Autodesk Inventor part; units mm, degrees
(part 2 of 3)
  line L944 (16.9524, -6.6944) -> (16.9314, -6.7061)
  line L945 (16.9314, -6.7061) -> (16.9218, -6.7147)
  line L946 (16.9218, -6.7147) -> (16.9143, -6.7266)
  line L947 (16.9143, -6.7266) -> (16.909, -6.7418)
  line L948 (16.909, -6.7418) -> (16.906, -6.76)
  line L949 (16.906, -6.76) -> (16.9054, -6.7813)
  line L950 (16.9054, -6.7813) -> (16.9073, -6.8056)
  line L951 (16.9073, -6.8056) -> (16.912, -6.8327)
  line L952 (16.912, -6.8327) -> (16.9194, -6.8625)
  line L953 (16.9194, -6.8625) -> (16.9472, -6.9448)
  line L954 (16.9472, -6.9448) -> (16.9649, -7.0024)
  line L955 (16.9649, -7.0024) -> (16.9847, -7.0784)
  line L956 (16.9847, -7.0784) -> (17.0036, -7.1659)
  line L957 (17.0036, -7.1659) -> (17.0214, -7.2683)
  line L958 (17.0214, -7.2683) -> (17.0364, -7.3838)
  line L959 (17.0364, -7.3838) -> (17.0479, -7.5139)
  line L960 (17.0479, -7.5139) -> (17.0545, -7.6588)
  line L961 (17.0545, -7.6588) -> (17.0557, -7.7357)
  line L962 (17.0557, -7.7357) -> (17.0536, -7.88)
  arc A25 (16.7145, -8.0349) -> (17.0536, -7.88) centre (13.25, 0) ccw
  line L963 (16.7145, -8.0349) -> (16.6041, -7.942)
  line L964 (16.6041, -7.942) -> (16.5467, -7.8907)
  line L965 (16.5467, -7.8907) -> (16.4415, -7.7908)
  line L966 (16.4415, -7.7908) -> (16.3508, -7.697)
  line L967 (16.3508, -7.697) -> (16.2733, -7.6099)
  line L968 (16.2733, -7.6099) -> (16.2075, -7.5295)
  line L969 (16.2075, -7.5295) -> (16.1538, -7.4579)
  line L970 (16.1538, -7.4579) -> (16.1094, -7.3931)
  line L971 (16.1094, -7.3931) -> (16.0773, -7.342)
  line L972 (16.0773, -7.342) -> (16.0334, -7.2672)
  line L973 (16.0334, -7.2672) -> (16.0157, -7.242)
  line L974 (16.0157, -7.242) -> (15.9983, -7.2207)
  line L975 (15.9983, -7.2207) -> (15.9812, -7.2034)
  line L976 (15.9812, -7.2034) -> (15.9647, -7.1899)
  line L977 (15.9647, -7.1899) -> (15.949, -7.1802)
  line L978 (15.949, -7.1802) -> (15.934, -7.1743)
  line L979 (15.934, -7.1743) -> (15.9201, -7.1722)
  line L980 (15.9201, -7.1722) -> (15.9073, -7.1738)
  line L981 (15.9073, -7.1738) -> (15.8847, -7.182)
  line L982 (15.8847, -7.182) -> (15.7521, -7.2293)
  line L983 (15.7521, -7.2293) -> (15.6186, -7.2741)
  line L984 (15.6186, -7.2741) -> (15.5957, -7.2816)
  line L985 (15.5957, -7.2816) -> (15.5847, -7.2883)
  line L986 (15.5847, -7.2883) -> (15.5751, -7.2986)
  line L987 (15.5751, -7.2986) -> (15.567, -7.3124)
  line L988 (15.567, -7.3124) -> (15.5605, -7.3298)
  line L989 (15.5605, -7.3298) -> (15.5559, -7.3506)
  line L990 (15.5559, -7.3506) -> (15.5533, -7.3747)
  line L991 (15.5533, -7.3747) -> (15.5527, -7.4022)
  line L992 (15.5527, -7.4022) -> (15.5544, -7.433)
  line L993 (15.5544, -7.433) -> (15.5661, -7.519)
  line L994 (15.5661, -7.519) -> (15.5725, -7.5789)
  line L995 (15.5725, -7.5789) -> (15.5776, -7.6573)
  line L996 (15.5776, -7.6573) -> (15.5796, -7.7468)
  line L997 (15.5796, -7.7468) -> (15.5777, -7.8506)
  line L998 (15.5777, -7.8506) -> (15.5706, -7.967)
  line L999 (15.5706, -7.967) -> (15.5572, -8.0968)
  line L1000 (15.5572, -8.0968) -> (15.5364, -8.2404)
  line L1001 (15.5364, -8.2404) -> (15.5229, -8.3162)
  line L1002 (15.5229, -8.3162) -> (15.4935, -8.4575)
  arc A26 (15.1313, -8.5454) -> (15.4935, -8.4575) centre (13.25, 0) ccw
  line L1003 (15.1313, -8.5454) -> (15.0404, -8.4332)
  line L1004 (15.0404, -8.4332) -> (14.9938, -8.372)
  line L1005 (14.9938, -8.372) -> (14.9094, -8.254)
  line L1006 (14.9094, -8.254) -> (14.8381, -8.1447)
  line L1007 (14.8381, -8.1447) -> (14.7785, -8.0445)
  line L1008 (14.7785, -8.0445) -> (14.7291, -7.9531)
  line L1009 (14.7291, -7.9531) -> (14.6899, -7.8727)
  line L1010 (14.6899, -7.8727) -> (14.6585, -7.8006)
  line L1011 (14.6585, -7.8006) -> (14.6368, -7.7444)
  line L1012 (14.6368, -7.7444) -> (14.6078, -7.6626)
  line L1013 (14.6078, -7.6626) -> (14.5952, -7.6345)
  line L1014 (14.5952, -7.6345) -> (14.5821, -7.6104)
  line L1015 (14.5821, -7.6104) -> (14.5686, -7.5901)
  line L1016 (14.5686, -7.5901) -> (14.555, -7.5737)
  line L1017 (14.555, -7.5737) -> (14.5413, -7.5612)
  line L1018 (14.5413, -7.5612) -> (14.5278, -7.5526)
  line L1019 (14.5278, -7.5526) -> (14.5145, -7.5479)
  line L1020 (14.5145, -7.5479) -> (14.5017, -7.547)
  line L1021 (14.5017, -7.547) -> (14.4779, -7.5508)
  line L1022 (14.4779, -7.5508) -> (14.3387, -7.5721)
  line L1023 (14.3387, -7.5721) -> (14.1992, -7.5909)
  line L1024 (14.1992, -7.5909) -> (14.1753, -7.594)
  line L1025 (14.1753, -7.594) -> (14.1632, -7.5984)
  line L1026 (14.1632, -7.5984) -> (14.1518, -7.6067)
  line L1027 (14.1518, -7.6067) -> (14.1412, -7.6187)
  line L1028 (14.1412, -7.6187) -> (14.1316, -7.6346)
  line L1029 (14.1316, -7.6346) -> (14.1232, -7.6541)
  line L1030 (14.1232, -7.6541) -> (14.116, -7.6774)
  line L1031 (14.116, -7.6774) -> (14.1102, -7.7043)
  line L1032 (14.1102, -7.7043) -> (14.106, -7.7347)
  line L1033 (14.106, -7.7347) -> (14.1013, -7.8214)
  line L1034 (14.1013, -7.8214) -> (14.0962, -7.8815)
  line L1035 (14.0962, -7.8815) -> (14.0864, -7.9594)
  line L1036 (14.0864, -7.9594) -> (14.0714, -8.0477)
  line L1037 (14.0714, -8.0477) -> (14.0499, -8.1493)
  line L1038 (14.0499, -8.1493) -> (14.0209, -8.2622)
  line L1039 (14.0209, -8.2622) -> (13.9832, -8.3872)
  line L1040 (13.9832, -8.3872) -> (13.9355, -8.5242)
  line L1041 (13.9355, -8.5242) -> (13.908, -8.5961)
  line L1042 (13.908, -8.5961) -> (13.8524, -8.7292)
  arc A27 (13.4801, -8.747) -> (13.8524, -8.7292) centre (13.25, 0) ccw
  line L1043 (13.4801, -8.747) -> (13.4121, -8.6197)
  line L1044 (13.4121, -8.6197) -> (13.3778, -8.5507)
  line L1045 (13.3778, -8.5507) -> (13.3174, -8.4189)
  line L1046 (13.3174, -8.4189) -> (13.268, -8.2981)
  line L1047 (13.268, -8.2981) -> (13.2284, -8.1884)
  line L1048 (13.2284, -8.1884) -> (13.1973, -8.0893)
  line L1049 (13.1973, -8.0893) -> (13.174, -8.0029)
  line L1050 (13.174, -8.0029) -> (13.1568, -7.9262)
  line L1051 (13.1568, -7.9262) -> (13.1461, -7.8669)
  line L1052 (13.1461, -7.8669) -> (13.1331, -7.7811)
  line L1053 (13.1331, -7.7811) -> (13.126, -7.7511)
  line L1054 (13.126, -7.7511) -> (13.1177, -7.7249)
  line L1055 (13.1177, -7.7249) -> (13.1084, -7.7025)
  line L1056 (13.1084, -7.7025) -> (13.0981, -7.6838)
  line L1057 (13.0981, -7.6838) -> (13.087, -7.669)
  line L1058 (13.087, -7.669) -> (13.0753, -7.658)
  line L1059 (13.0753, -7.658) -> (13.0632, -7.6508)
  line L1060 (13.0632, -7.6508) -> (13.0508, -7.6475)
  line L1061 (13.0508, -7.6475) -> (13.0267, -7.6468)
  line L1062 (13.0267, -7.6468) -> (12.886, -7.6413)
  line L1063 (12.886, -7.6413) -> (12.7454, -7.6334)
  line L1064 (12.7454, -7.6334) -> (12.7214, -7.6318)
  line L1065 (12.7214, -7.6318) -> (12.7087, -7.6339)
  line L1066 (12.7087, -7.6339) -> (12.6959, -7.6399)
  line L1067 (12.6959, -7.6399) -> (12.6833, -7.6497)
  line L1068 (12.6833, -7.6497) -> (12.6708, -7.6635)
  line L1069 (12.6708, -7.6635) -> (12.6588, -7.6811)
  line L1070 (12.6588, -7.6811) -> (12.6474, -7.7025)
  line L1071 (12.6474, -7.7025) -> (12.6366, -7.7278)
  line L1072 (12.6366, -7.7278) -> (12.6267, -7.757)
  line L1073 (12.6267, -7.757) -> (12.6057, -7.8412)
  line L1074 (12.6057, -7.8412) -> (12.5893, -7.8992)
  line L1075 (12.5893, -7.8992) -> (12.5649, -7.9739)
  line L1076 (12.5649, -7.9739) -> (12.5336, -8.0577)
  line L1077 (12.5336, -8.0577) -> (12.4931, -8.1534)
  line L1078 (12.4931, -8.1534) -> (12.4433, -8.2588)
  line L1079 (12.4433, -8.2588) -> (12.3827, -8.3744)
  line L1080 (12.3827, -8.3744) -> (12.3099, -8.4999)
  line L1081 (12.3099, -8.4999) -> (12.2693, -8.5652)
  line L1082 (12.2693, -8.5652) -> (12.1895, -8.6855)
  arc A28 (11.8205, -8.6324) -> (12.1895, -8.6855) centre (13.25, 0) ccw
  line L1083 (11.8205, -8.6324) -> (11.7779, -8.4946)
  line L1084 (11.7779, -8.4946) -> (11.7573, -8.4204)
  line L1085 (11.7573, -8.4204) -> (11.7229, -8.2795)
  line L1086 (11.7229, -8.2795) -> (11.6972, -8.1515)
  line L1087 (11.6972, -8.1515) -> (11.6791, -8.0364)
  line L1088 (11.6791, -8.0364) -> (11.6673, -7.9332)
  line L1089 (11.6673, -7.9332) -> (11.6608, -7.8439)
  line L1090 (11.6608, -7.8439) -> (11.6584, -7.7654)
  line L1091 (11.6584, -7.7654) -> (11.6591, -7.7051)
  line L1092 (11.6591, -7.7051) -> (11.6626, -7.6183)
  line L1093 (11.6626, -7.6183) -> (11.6614, -7.5876)
  line L1094 (11.6614, -7.5876) -> (11.6582, -7.5603)
  line L1095 (11.6582, -7.5603) -> (11.6532, -7.5365)
  line L1096 (11.6532, -7.5365) -> (11.6467, -7.5162)
  line L1097 (11.6467, -7.5162) -> (11.6386, -7.4995)
  line L1098 (11.6386, -7.4995) -> (11.6292, -7.4865)
  line L1099 (11.6292, -7.4865) -> (11.6187, -7.4772)
  line L1100 (11.6187, -7.4772) -> (11.6071, -7.4716)
  line L1101 (11.6071, -7.4716) -> (11.5836, -7.4663)
  line L1102 (11.5836, -7.4663) -> (11.4464, -7.4344)
  line L1103 (11.4464, -7.4344) -> (11.3099, -7.3999)
  line L1104 (11.3099, -7.3999) -> (11.2866, -7.3939)
  line L1105 (11.2866, -7.3939) -> (11.2737, -7.3935)
  line L1106 (11.2737, -7.3935) -> (11.2601, -7.397)
  line L1107 (11.2601, -7.397) -> (11.2458, -7.4042)
  line L1108 (11.2458, -7.4042) -> (11.231, -7.4154)
  line L1109 (11.231, -7.4154) -> (11.2159, -7.4304)
  line L1110 (11.2159, -7.4304) -> (11.2005, -7.4493)
  line L1111 (11.2005, -7.4493) -> (11.1852, -7.4721)
  line L1112 (11.1852, -7.4721) -> (11.17, -7.4988)
  line L1113 (11.17, -7.4988) -> (11.1334, -7.5775)
  line L1114 (11.1334, -7.5775) -> (11.1063, -7.6314)
  line L1115 (11.1063, -7.6314) -> (11.0683, -7.7001)
  line L1116 (11.0683, -7.7001) -> (11.0216, -7.7765)
  line L1117 (11.0216, -7.7765) -> (10.9638, -7.8628)
  line L1118 (10.9638, -7.8628) -> (10.8949, -7.9569)
  line L1119 (10.8949, -7.9569) -> (10.8135, -8.0589)
  line L1120 (10.8135, -8.0589) -> (10.7183, -8.1683)
  line L1121 (10.7183, -8.1683) -> (10.666, -8.2249)
  line L1122 (10.666, -8.2249) -> (10.5649, -8.3278)
  arc A29 (10.2127, -8.2059) -> (10.5649, -8.3278) centre (13.25, 0) ccw
  line L1123 (10.2127, -8.2059) -> (10.1969, -8.0625)
  line L1124 (10.1969, -8.0625) -> (10.1907, -7.9857)
  line L1125 (10.1907, -7.9857) -> (10.1836, -7.8409)
  line L1126 (10.1836, -7.8409) -> (10.1826, -7.7103)
  line L1127 (10.1826, -7.7103) -> (10.1866, -7.5938)
  line L1128 (10.1866, -7.5938) -> (10.1945, -7.4903)
  line L1129 (10.1945, -7.4903) -> (10.2051, -7.4014)
  line L1130 (10.2051, -7.4014) -> (10.2176, -7.3238)
  line L1131 (10.2176, -7.3238) -> (10.2297, -7.2647)
  line L1132 (10.2297, -7.2647) -> (10.2495, -7.1803)
  line L1133 (10.2495, -7.1803) -> (10.2541, -7.1498)
  line L1134 (10.2541, -7.1498) -> (10.2561, -7.1224)
  line L1135 (10.2561, -7.1224) -> (10.2558, -7.0981)
  line L1136 (10.2558, -7.0981) -> (10.2532, -7.0769)
  line L1137 (10.2532, -7.0769) -> (10.2484, -7.059)
  line L1138 (10.2484, -7.059) -> (10.2417, -7.0445)
  line L1139 (10.2417, -7.0445) -> (10.2331, -7.0333)
  line L1140 (10.2331, -7.0333) -> (10.2227, -7.0257)
  line L1141 (10.2227, -7.0257) -> (10.2007, -7.016)
  line L1142 (10.2007, -7.016) -> (10.0721, -6.9587)
  line L1143 (10.0721, -6.9587) -> (9.9445, -6.899)
  line L1144 (9.9445, -6.899) -> (9.9228, -6.8887)
  line L1145 (9.9228, -6.8887) -> (9.9102, -6.8859)
  line L1146 (9.9102, -6.8859) -> (9.8962, -6.8867)
  line L1147 (9.8962, -6.8867) -> (9.8807, -6.8911)
  line L1148 (9.8807, -6.8911) -> (9.8641, -6.8993)
  line L1149 (9.8641, -6.8993) -> (9.8464, -6.9111)
  line L1150 (9.8464, -6.9111) -> (9.8278, -6.9268)
  line L1151 (9.8278, -6.9268) -> (9.8084, -6.9463)
  line L1152 (9.8084, -6.9463) -> (9.7884, -6.9697)
  line L1153 (9.7884, -6.9697) -> (9.7376, -7.04)
  line L1154 (9.7376, -7.04) -> (9.7008, -7.0878)
  line L1155 (9.7008, -7.0878) -> (9.6504, -7.1481)
  line L1156 (9.6504, -7.1481) -> (9.5901, -7.2143)
  line L1157 (9.5901, -7.2143) -> (9.5171, -7.2881)
  line L1158 (9.5171, -7.2881) -> (9.4316, -7.3674)
  line L1159 (9.4316, -7.3674) -> (9.3324, -7.4521)
  line L1160 (9.3324, -7.4521) -> (9.2182, -7.5416)
  line L1161 (9.2182, -7.5416) -> (9.1562, -7.5872)
  line L1162 (9.1562, -7.5872) -> (9.0374, -7.6692)
  arc A30 (8.7146, -7.4828) -> (9.0374, -7.6692) centre (13.25, 0) ccw
  line L1163 (8.7146, -7.4828) -> (8.7262, -7.339)
  line L1164 (8.7262, -7.339) -> (8.7347, -7.2624)
  line L1165 (8.7347, -7.2624) -> (8.7551, -7.1188)
  line L1166 (8.7551, -7.1188) -> (8.7788, -6.9905)
  line L1167 (8.7788, -6.9905) -> (8.8048, -6.8769)
  line L1168 (8.8048, -6.8769) -> (8.8322, -6.7767)
  line L1169 (8.8322, -6.7767) -> (8.8594, -6.6914)
  line L1170 (8.8594, -6.6914) -> (8.8863, -6.6176)
  line L1171 (8.8863, -6.6176) -> (8.9094, -6.5619)
  line L1172 (8.9094, -6.5619) -> (8.9449, -6.4827)
  line L1173 (8.9449, -6.4827) -> (8.9551, -6.4536)
  line L1174 (8.9551, -6.4536) -> (8.9623, -6.4271)
  line L1175 (8.9623, -6.4271) -> (8.9666, -6.4032)
  line L1176 (8.9666, -6.4032) -> (8.968, -6.3819)
  line L1177 (8.968, -6.3819) -> (8.9667, -6.3634)
  line L1178 (8.9667, -6.3634) -> (8.9629, -6.3479)
  line L1179 (8.9629, -6.3479) -> (8.9565, -6.3353)
  line L1180 (8.9565, -6.3353) -> (8.9478, -6.3258)
  line L1181 (8.9478, -6.3258) -> (8.928, -6.3121)
  line L1182 (8.928, -6.3121) -> (8.8126, -6.2315)
  line L1183 (8.8126, -6.2315) -> (8.6986, -6.1488)
  line L1184 (8.6986, -6.1488) -> (8.6792, -6.1345)
  line L1185 (8.6792, -6.1345) -> (8.6674, -6.1294)
  line L1186 (8.6674, -6.1294) -> (8.6535, -6.1275)
  line L1187 (8.6535, -6.1275) -> (8.6375, -6.129)
  line L1188 (8.6375, -6.129) -> (8.6196, -6.1338)
  line L1189 (8.6196, -6.1338) -> (8.6, -6.1421)
  line L1190 (8.6, -6.1421) -> (8.5787, -6.154)
  line L1191 (8.5787, -6.154) -> (8.556, -6.1694)
  line L1192 (8.556, -6.1694) -> (8.532, -6.1886)
  line L1193 (8.532, -6.1886) -> (8.4687, -6.248)
  line L1194 (8.4687, -6.248) -> (8.4236, -6.2881)
  line L1195 (8.4236, -6.2881) -> (8.3627, -6.3377)
  line L1196 (8.3627, -6.3377) -> (8.291, -6.3913)
  line L1197 (8.291, -6.3913) -> (8.2052, -6.4499)
  line L1198 (8.2052, -6.4499) -> (8.1063, -6.5116)
  line L1199 (8.1063, -6.5116) -> (7.9928, -6.576)
  line L1200 (7.9928, -6.576) -> (7.8638, -6.6423)
  line L1201 (7.8638, -6.6423) -> (7.7943, -6.6753)
  line L1202 (7.7943, -6.6753) -> (7.6621, -6.7334)
  arc A31 (7.3804, -6.4893) -> (7.6621, -6.7334) centre (13.25, 0) ccw
  line L1203 (7.3804, -6.4893) -> (7.4191, -6.3502)
  line L1204 (7.4191, -6.3502) -> (7.4418, -6.2767)
  line L1205 (7.4418, -6.2767) -> (7.4891, -6.1395)
  line L1206 (7.4891, -6.1395) -> (7.5367, -6.018)
  line L1207 (7.5367, -6.018) -> (7.5837, -5.9113)
  line L1208 (7.5837, -5.9113) -> (7.6295, -5.8181)
  line L1209 (7.6295, -5.8181) -> (7.6724, -5.7395)
  line L1210 (7.6724, -5.7395) -> (7.7128, -5.6722)
  line L1211 (7.7128, -5.6722) -> (7.746, -5.6218)
  line L1212 (7.746, -5.6218) -> (7.7958, -5.5508)
  line L1213 (7.7958, -5.5508) -> (7.8114, -5.5242)
  line L1214 (7.8114, -5.5242) -> (7.8235, -5.4995)
  line L1215 (7.8235, -5.4995) -> (7.8322, -5.4768)
  line L1216 (7.8322, -5.4768) -> (7.8376, -5.4562)
  line L1217 (7.8376, -5.4562) -> (7.8399, -5.4378)
  line L1218 (7.8399, -5.4378) -> (7.839, -5.4218)
  line L1219 (7.839, -5.4218) -> (7.8352, -5.4082)
  line L1220 (7.8352, -5.4082) -> (7.8284, -5.3973)
  line L1221 (7.8284, -5.3973) -> (7.8115, -5.3801)
  line L1222 (7.8115, -5.3801) -> (7.7134, -5.2791)
  line L1223 (7.7134, -5.2791) -> (7.6172, -5.1763)
  line L1224 (7.6172, -5.1763) -> (7.6008, -5.1586)
  line L1225 (7.6008, -5.1586) -> (7.5902, -5.1514)
  line L1226 (7.5902, -5.1514) -> (7.5769, -5.1469)
  line L1227 (7.5769, -5.1469) -> (7.5609, -5.1453)
  line L1228 (7.5609, -5.1453) -> (7.5424, -5.1466)
  line L1229 (7.5424, -5.1466) -> (7.5216, -5.1511)
  line L1230 (7.5216, -5.1511) -> (7.4985, -5.1587)
  line L1231 (7.4985, -5.1587) -> (7.4733, -5.1696)
  line L1232 (7.4733, -5.1696) -> (7.446, -5.1839)
  line L1233 (7.446, -5.1839) -> (7.3727, -5.2303)
  line L1234 (7.3727, -5.2303) -> (7.3208, -5.261)
  line L1235 (7.3208, -5.261) -> (7.2516, -5.2982)
  line L1236 (7.2516, -5.2982) -> (7.171, -5.3373)
  line L1237 (7.171, -5.3373) -> (7.0758, -5.3786)
  line L1238 (7.0758, -5.3786) -> (6.967, -5.4205)
  line L1239 (6.967, -5.4205) -> (6.8433, -5.4623)
  line L1240 (6.8433, -5.4623) -> (6.7041, -5.5029)
  line L1241 (6.7041, -5.5029) -> (6.6295, -5.5222)
  line L1242 (6.6295, -5.5222) -> (6.4888, -5.5542)
  arc A32 (6.2584, -5.2612) -> (6.4888, -5.5542) centre (13.25, 0) ccw
  line L1243 (6.2584, -5.2612) -> (6.3226, -5.1319)
  line L1244 (6.3226, -5.1319) -> (6.3589, -5.064)
  line L1245 (6.3589, -5.064) -> (6.4313, -4.9383)
  line L1246 (6.4313, -4.9383) -> (6.501, -4.828)
  line L1247 (6.501, -4.828) -> (6.5674, -4.7321)
  line L1248 (6.5674, -4.7321) -> (6.63, -4.6493)
  line L1249 (6.63, -4.6493) -> (6.6869, -4.5802)
  line L1250 (6.6869, -4.5802) -> (6.7394, -4.5218)
  line L1251 (6.7394, -4.5218) -> (6.7815, -4.4786)
  line L1252 (6.7815, -4.4786) -> (6.8439, -4.4182)
  line L1253 (6.8439, -4.4182) -> (6.8642, -4.3951)
  line L1254 (6.8642, -4.3951) -> (6.8807, -4.3732)
  line L1255 (6.8807, -4.3732) -> (6.8936, -4.3525)
  line L1256 (6.8936, -4.3525) -> (6.9028, -4.3333)
  line L1257 (6.9028, -4.3333) -> (6.9085, -4.3157)
  line L1258 (6.9085, -4.3157) -> (6.9107, -4.2998)
  line L1259 (6.9107, -4.2998) -> (6.9095, -4.2857)
  line L1260 (6.9095, -4.2857) -> (6.9049, -4.2737)
  line L1261 (6.9049, -4.2737) -> (6.8916, -4.2537)
  line L1262 (6.8916, -4.2537) -> (6.8144, -4.1359)
  line L1263 (6.8144, -4.1359) -> (6.7394, -4.0168)
  line L1264 (6.7394, -4.0168) -> (6.7267, -3.9963)
  line L1265 (6.7267, -3.9963) -> (6.7176, -3.9872)
  line L1266 (6.7176, -3.9872) -> (6.7053, -3.9802)
  line L1267 (6.7053, -3.9802) -> (6.69, -3.9756)
  line L1268 (6.69, -3.9756) -> (6.6716, -3.9735)
  line L1269 (6.6716, -3.9735) -> (6.6503, -3.9739)
  line L1270 (6.6503, -3.9739) -> (6.6262, -3.977)
  line L1271 (6.6262, -3.977) -> (6.5993, -3.9829)
  line L1272 (6.5993, -3.9829) -> (6.5698, -3.9918)
  line L1273 (6.5698, -3.9918) -> (6.489, -4.0235)
  line L1274 (6.489, -4.0235) -> (6.4323, -4.0438)
  line L1275 (6.4323, -4.0438) -> (6.3573, -4.0673)
  line L1276 (6.3573, -4.0673) -> (6.2708, -4.0904)
  line L1277 (6.2708, -4.0904) -> (6.1694, -4.1129)
  line L1278 (6.1694, -4.1129) -> (6.0547, -4.1335)
  line L1279 (6.0547, -4.1335) -> (5.9254, -4.1511)
  line L1280 (5.9254, -4.1511) -> (5.7809, -4.1647)
  line L1281 (5.7809, -4.1647) -> (5.7041, -4.1695)
  line L1282 (5.7041, -4.1695) -> (5.5599, -4.1742)
  arc A33 (5.3891, -3.8429) -> (5.5599, -4.1742) centre (13.25, 0) ccw
  line L1283 (5.3891, -3.8429) -> (5.4766, -3.7282)
  line L1284 (5.4766, -3.7282) -> (5.5251, -3.6684)
  line L1285 (5.5251, -3.6684) -> (5.6199, -3.5586)
  line L1286 (5.6199, -3.5586) -> (5.7093, -3.4635)
  line L1287 (5.7093, -3.4635) -> (5.7926, -3.3819)
  line L1288 (5.7926, -3.3819) -> (5.8698, -3.3125)
  line L1289 (5.8698, -3.3125) -> (5.9387, -3.2554)
  line L1290 (5.9387, -3.2554) -> (6.0013, -3.2079)
  line L1291 (6.0013, -3.2079) -> (6.0508, -3.1735)
  line L1292 (6.0508, -3.1735) -> (6.1235, -3.126)
  line L1293 (6.1235, -3.126) -> (6.1478, -3.1072)
  line L1294 (6.1478, -3.1072) -> (6.1682, -3.0887)
  line L1295 (6.1682, -3.0887) -> (6.1847, -3.0709)
  line L1296 (6.1847, -3.0709) -> (6.1974, -3.0538)
  line L1297 (6.1974, -3.0538) -> (6.2064, -3.0375)
  line L1298 (6.2064, -3.0375) -> (6.2115, -3.0223)
  line L1299 (6.2115, -3.0223) -> (6.213, -3.0083)
  line L1300 (6.213, -3.0083) -> (6.2108, -2.9957)
  line L1301 (6.2108, -2.9957) -> (6.2015, -2.9735)
  line L1302 (6.2015, -2.9735) -> (6.148, -2.8432)
  line L1303 (6.148, -2.8432) -> (6.0968, -2.712)
  line L1304 (6.0968, -2.712) -> (6.0882, -2.6895)
  line L1305 (6.0882, -2.6895) -> (6.0811, -2.6789)
  line L1306 (6.0811, -2.6789) -> (6.0703, -2.6697)
  line L1307 (6.0703, -2.6697) -> (6.0561, -2.6623)
  line L1308 (6.0561, -2.6623) -> (6.0385, -2.6567)
  line L1309 (6.0385, -2.6567) -> (6.0175, -2.6531)
  line L1310 (6.0175, -2.6531) -> (5.9932, -2.6516)
  line L1311 (5.9932, -2.6516) -> (5.9657, -2.6523)
  line L1312 (5.9657, -2.6523) -> (5.9351, -2.6554)
  line L1313 (5.9351, -2.6554) -> (5.8498, -2.6712)
  line L1314 (5.8498, -2.6712) -> (5.7902, -2.6805)
  line L1315 (5.7902, -2.6805) -> (5.7121, -2.6893)
  line L1316 (5.7121, -2.6893) -> (5.6228, -2.6956)
  line L1317 (5.6228, -2.6956) -> (5.519, -2.6986)
  line L1318 (5.519, -2.6986) -> (5.4024, -2.697)
  line L1319 (5.4024, -2.697) -> (5.2721, -2.6899)
  line L1320 (5.2721, -2.6899) -> (5.1277, -2.6759)
  line L1321 (5.1277, -2.6759) -> (5.0514, -2.666)
  line L1322 (5.0514, -2.666) -> (4.9089, -2.6434)
  arc A34 (4.8038, -2.2858) -> (4.9089, -2.6434) centre (13.25, 0) ccw
  line L1323 (4.8038, -2.2858) -> (4.9115, -2.1897)
  line L1324 (4.9115, -2.1897) -> (4.9704, -2.1401)
  line L1325 (4.9704, -2.1401) -> (5.0843, -2.0503)
  line L1326 (5.0843, -2.0503) -> (5.1901, -1.9738)
  line L1327 (5.1901, -1.9738) -> (5.2873, -1.9095)
  line L1328 (5.2873, -1.9095) -> (5.3762, -1.8559)
  line L1329 (5.3762, -1.8559) -> (5.4548, -1.8129)
  line L1330 (5.4548, -1.8129) -> (5.5252, -1.7781)
  line L1331 (5.5252, -1.7781) -> (5.5804, -1.7537)
  line L1332 (5.5804, -1.7537) -> (5.6607, -1.7208)
  line L1333 (5.6607, -1.7208) -> (5.6881, -1.7069)
  line L1334 (5.6881, -1.7069) -> (5.7116, -1.6927)
  line L1335 (5.7116, -1.6927) -> (5.7313, -1.6783)
  line L1336 (5.7313, -1.6783) -> (5.747, -1.6639)
  line L1337 (5.747, -1.6639) -> (5.7588, -1.6496)
  line L1338 (5.7588, -1.6496) -> (5.7667, -1.6357)
  line L1339 (5.7667, -1.6357) -> (5.7708, -1.6222)
  line L1340 (5.7708, -1.6222) -> (5.7711, -1.6094)
  line L1341 (5.7711, -1.6094) -> (5.7661, -1.5858)
  line L1342 (5.7661, -1.5858) -> (5.7382, -1.4478)
  line L1343 (5.7382, -1.4478) -> (5.7128, -1.3093)
  line L1344 (5.7128, -1.3093) -> (5.7087, -1.2856)
  line L1345 (5.7087, -1.2856) -> (5.7036, -1.2737)
  line L1346 (5.7036, -1.2737) -> (5.6948, -1.2627)
  line L1347 (5.6948, -1.2627) -> (5.6823, -1.2527)
  line L1348 (5.6823, -1.2527) -> (5.666, -1.2439)
  line L1349 (5.666, -1.2439) -> (5.6461, -1.2364)
  line L1350 (5.6461, -1.2364) -> (5.6225, -1.2303)
  line L1351 (5.6225, -1.2303) -> (5.5954, -1.2258)
  line L1352 (5.5954, -1.2258) -> (5.5648, -1.2231)
  line L1353 (5.5648, -1.2231) -> (5.478, -1.2224)
  line L1354 (5.478, -1.2224) -> (5.4177, -1.2203)
  line L1355 (5.4177, -1.2203) -> (5.3394, -1.2142)
  line L1356 (5.3394, -1.2142) -> (5.2505, -1.2034)
  line L1357 (5.2505, -1.2034) -> (5.148, -1.1867)
  line L1358 (5.148, -1.1867) -> (5.0338, -1.1631)
  line L1359 (5.0338, -1.1631) -> (4.9072, -1.1315)
  line L1360 (4.9072, -1.1315) -> (4.7681, -1.0904)
  line L1361 (4.7681, -1.0904) -> (4.695, -1.0663)
  line L1362 (4.695, -1.0663) -> (4.5593, -1.0171)
  arc A35 (4.5239, -0.646) -> (4.5593, -1.0171) centre (13.25, 0) ccw
  line L1363 (4.5239, -0.646) -> (4.6478, -0.572)
  line L1364 (4.6478, -0.572) -> (4.715, -0.5346)
  line L1365 (4.715, -0.5346) -> (4.8439, -0.4679)
  line L1366 (4.8439, -0.4679) -> (4.9622, -0.4128)
  line L1367 (4.9622, -0.4128) -> (5.0698, -0.368)
  line L1368 (5.0698, -0.368) -> (5.1673, -0.3322)
  line L1369 (5.1673, -0.3322) -> (5.2526, -0.3049)
  line L1370 (5.2526, -0.3049) -> (5.3283, -0.2841)
  line L1371 (5.3283, -0.2841) -> (5.3871, -0.2705)
  line L1372 (5.3871, -0.2705) -> (5.4722, -0.2535)
  line L1373 (5.4722, -0.2535) -> (5.5017, -0.245)
  line L1374 (5.5017, -0.245) -> (5.5275, -0.2354)
  line L1375 (5.5275, -0.2354) -> (5.5495, -0.225)
  line L1376 (5.5495, -0.225) -> (5.5677, -0.2139)
  line L1377 (5.5677, -0.2139) -> (5.582, -0.2021)
  line L1378 (5.582, -0.2021) -> (5.5924, -0.1899)
  line L1379 (5.5924, -0.1899) -> (5.599, -0.1775)
  line L1380 (5.599, -0.1775) -> (5.6017, -0.1649)
  line L1381 (5.6017, -0.1649) -> (5.6013, -0.1408)
  line L1382 (5.6013, -0.1408) -> (5.6, 0)
  line L1383 (5.6, 0) -> (5.6013, 0.1408)
  line L1384 (5.6013, 0.1408) -> (5.6017, 0.1649)
  line L1385 (5.6017, 0.1649) -> (5.599, 0.1775)
  line L1386 (5.599, 0.1775) -> (5.5924, 0.1899)
  line L1387 (5.5924, 0.1899) -> (5.582, 0.2021)
  line L1388 (5.582, 0.2021) -> (5.5677, 0.2139)
  line L1389 (5.5677, 0.2139) -> (5.5495, 0.225)
  line L1390 (5.5495, 0.225) -> (5.5275, 0.2354)
  line L1391 (5.5275, 0.2354) -> (5.5017, 0.245)
  line L1392 (5.5017, 0.245) -> (5.4722, 0.2535)
  line L1393 (5.4722, 0.2535) -> (5.3871, 0.2705)
  line L1394 (5.3871, 0.2705) -> (5.3283, 0.2841)
  line L1395 (5.3283, 0.2841) -> (5.2526, 0.3049)
  line L1396 (5.2526, 0.3049) -> (5.1673, 0.3322)
  line L1397 (5.1673, 0.3322) -> (5.0698, 0.368)
  line L1398 (5.0698, 0.368) -> (4.9622, 0.4128)
  line L1399 (4.9622, 0.4128) -> (4.8439, 0.4679)
  line L1400 (4.8439, 0.4679) -> (4.715, 0.5346)
  line L1401 (4.715, 0.5346) -> (4.6478, 0.572)
  line L1402 (4.6478, 0.572) -> (4.5239, 0.646)
  arc A36 (4.5593, 1.0171) -> (4.5239, 0.646) centre (13.25, 0) ccw
  line L1403 (4.5593, 1.0171) -> (4.695, 1.0663)
  line L1404 (4.695, 1.0663) -> (4.7681, 1.0904)
  line L1405 (4.7681, 1.0904) -> (4.9072, 1.1315)
  line L1406 (4.9072, 1.1315) -> (5.0338, 1.1631)
  line L1407 (5.0338, 1.1631) -> (5.148, 1.1867)
  line L1408 (5.148, 1.1867) -> (5.2505, 1.2034)
  line L1409 (5.2505, 1.2034) -> (5.3394, 1.2142)
  line L1410 (5.3394, 1.2142) -> (5.4177, 1.2203)
  line L1411 (5.4177, 1.2203) -> (5.478, 1.2224)
  line L1412 (5.478, 1.2224) -> (5.5648, 1.2231)
  line L1413 (5.5648, 1.2231) -> (5.5954, 1.2258)
  line L1414 (5.5954, 1.2258) -> (5.6225, 1.2303)
  line L1415 (5.6225, 1.2303) -> (5.6461, 1.2364)
  line L1416 (5.6461, 1.2364) -> (5.666, 1.2439)
  line L1417 (5.666, 1.2439) -> (5.6823, 1.2527)
  line L1418 (5.6823, 1.2527) -> (5.6948, 1.2627)
  line L1419 (5.6948, 1.2627) -> (5.7036, 1.2737)
  line L1420 (5.7036, 1.2737) -> (5.7087, 1.2856)
  line L1421 (5.7087, 1.2856) -> (5.7128, 1.3093)
  line L1422 (5.7128, 1.3093) -> (5.7382, 1.4478)
  line L1423 (5.7382, 1.4478) -> (5.7661, 1.5858)
  line L1424 (5.7661, 1.5858) -> (5.7711, 1.6094)
  line L1425 (5.7711, 1.6094) -> (5.7708, 1.6222)
  line L1426 (5.7708, 1.6222) -> (5.7667, 1.6357)
  line L1427 (5.7667, 1.6357) -> (5.7588, 1.6496)
  line L1428 (5.7588, 1.6496) -> (5.747, 1.6639)
  line L1429 (5.747, 1.6639) -> (5.7313, 1.6783)
  line L1430 (5.7313, 1.6783) -> (5.7116, 1.6927)
  line L1431 (5.7116, 1.6927) -> (5.6881, 1.7069)
  line L1432 (5.6881, 1.7069) -> (5.6607, 1.7208)
  line L1433 (5.6607, 1.7208) -> (5.5804, 1.7537)
  line L1434 (5.5804, 1.7537) -> (5.5252, 1.7781)
  line L1435 (5.5252, 1.7781) -> (5.4548, 1.8129)
  line L1436 (5.4548, 1.8129) -> (5.3762, 1.8559)
  line L1437 (5.3762, 1.8559) -> (5.2873, 1.9095)
  line L1438 (5.2873, 1.9095) -> (5.1901, 1.9738)
  line L1439 (5.1901, 1.9738) -> (5.0843, 2.0503)
  line L1440 (5.0843, 2.0503) -> (4.9704, 2.1401)
  line L1441 (4.9704, 2.1401) -> (4.9115, 2.1897)
  line L1442 (4.9115, 2.1897) -> (4.8038, 2.2858)
  arc A37 (4.9089, 2.6434) -> (4.8038, 2.2858) centre (13.25, 0) ccw
  line L1443 (4.9089, 2.6434) -> (5.0514, 2.666)
  line L1444 (5.0514, 2.666) -> (5.1277, 2.6759)
  line L1445 (5.1277, 2.6759) -> (5.2721, 2.6899)
  line L1446 (5.2721, 2.6899) -> (5.4024, 2.697)
  line L1447 (5.4024, 2.697) -> (5.519, 2.6986)
  line L1448 (5.519, 2.6986) -> (5.6228, 2.6956)
  line L1449 (5.6228, 2.6956) -> (5.7121, 2.6893)
  line L1450 (5.7121, 2.6893) -> (5.7902, 2.6805)
  line L1451 (5.7902, 2.6805) -> (5.8498, 2.6712)
  line L1452 (5.8498, 2.6712) -> (5.9351, 2.6554)
  line L1453 (5.9351, 2.6554) -> (5.9657, 2.6523)
  line L1454 (5.9657, 2.6523) -> (5.9932, 2.6516)
  line L1455 (5.9932, 2.6516) -> (6.0175, 2.6531)
  line L1456 (6.0175, 2.6531) -> (6.0385, 2.6567)
  line L1457 (6.0385, 2.6567) -> (6.0561, 2.6623)
  line L1458 (6.0561, 2.6623) -> (6.0703, 2.6697)
  line L1459 (6.0703, 2.6697) -> (6.0811, 2.6789)
  line L1460 (6.0811, 2.6789) -> (6.0882, 2.6895)
  line L1461 (6.0882, 2.6895) -> (6.0968, 2.712)
  line L1462 (6.0968, 2.712) -> (6.148, 2.8432)
  line L1463 (6.148, 2.8432) -> (6.2015, 2.9735)
  line L1464 (6.2015, 2.9735) -> (6.2108, 2.9957)
  line L1465 (6.2108, 2.9957) -> (6.213, 3.0083)
  line L1466 (6.213, 3.0083) -> (6.2115, 3.0223)
  line L1467 (6.2115, 3.0223) -> (6.2064, 3.0375)
  line L1468 (6.2064, 3.0375) -> (6.1974, 3.0538)
  line L1469 (6.1974, 3.0538) -> (6.1847, 3.0709)
  line L1470 (6.1847, 3.0709) -> (6.1682, 3.0887)
  line L1471 (6.1682, 3.0887) -> (6.1478, 3.1072)
  line L1472 (6.1478, 3.1072) -> (6.1235, 3.126)
  line L1473 (6.1235, 3.126) -> (6.0508, 3.1735)
  line L1474 (6.0508, 3.1735) -> (6.0013, 3.2079)
  line L1475 (6.0013, 3.2079) -> (5.9387, 3.2554)
  line L1476 (5.9387, 3.2554) -> (5.8698, 3.3125)
  line L1477 (5.8698, 3.3125) -> (5.7926, 3.3819)
  line L1478 (5.7926, 3.3819) -> (5.7093, 3.4635)
  line L1479 (5.7093, 3.4635) -> (5.6199, 3.5586)
  line L1480 (5.6199, 3.5586) -> (5.5251, 3.6684)
  line L1481 (5.5251, 3.6684) -> (5.4766, 3.7282)
  line L1482 (5.4766, 3.7282) -> (5.3891, 3.8429)
  arc A38 (5.5599, 4.1742) -> (5.3891, 3.8429) centre (13.25, 0) ccw
  line L1483 (5.5599, 4.1742) -> (5.7041, 4.1695)
  line L1484 (5.7041, 4.1695) -> (5.7809, 4.1647)
  line L1485 (5.7809, 4.1647) -> (5.9254, 4.1511)
  line L1486 (5.9254, 4.1511) -> (6.0547, 4.1335)
  line L1487 (6.0547, 4.1335) -> (6.1694, 4.1129)
  line L1488 (6.1694, 4.1129) -> (6.2708, 4.0904)
  line L1489 (6.2708, 4.0904) -> (6.3573, 4.0673)
  line L1490 (6.3573, 4.0673) -> (6.4323, 4.0438)
  line L1491 (6.4323, 4.0438) -> (6.489, 4.0235)
  line L1492 (6.489, 4.0235) -> (6.5698, 3.9918)
  line L1493 (6.5698, 3.9918) -> (6.5993, 3.9829)
  line L1494 (6.5993, 3.9829) -> (6.6262, 3.977)
  line L1495 (6.6262, 3.977) -> (6.6503, 3.9739)
  line L1496 (6.6503, 3.9739) -> (6.6716, 3.9735)
  line L1497 (6.6716, 3.9735) -> (6.69, 3.9756)
  line L1498 (6.69, 3.9756) -> (6.7053, 3.9802)
  line L1499 (6.7053, 3.9802) -> (6.7176, 3.9872)
  line L1500 (6.7176, 3.9872) -> (6.7267, 3.9963)
  line L1501 (6.7267, 3.9963) -> (6.7394, 4.0168)
  line L1502 (6.7394, 4.0168) -> (6.8144, 4.1359)
  line L1503 (6.8144, 4.1359) -> (6.8916, 4.2537)
  line L1504 (6.8916, 4.2537) -> (6.9049, 4.2737)
  line L1505 (6.9049, 4.2737) -> (6.9095, 4.2857)
  line L1506 (6.9095, 4.2857) -> (6.9107, 4.2998)
  line L1507 (6.9107, 4.2998) -> (6.9085, 4.3157)
  line L1508 (6.9085, 4.3157) -> (6.9028, 4.3333)
  line L1509 (6.9028, 4.3333) -> (6.8936, 4.3525)
  line L1510 (6.8936, 4.3525) -> (6.8807, 4.3732)
  line L1511 (6.8807, 4.3732) -> (6.8642, 4.3951)
  line L1512 (6.8642, 4.3951) -> (6.8439, 4.4182)
  line L1513 (6.8439, 4.4182) -> (6.7815, 4.4786)
  line L1514 (6.7815, 4.4786) -> (6.7394, 4.5218)
  line L1515 (6.7394, 4.5218) -> (6.6869, 4.5802)
  line L1516 (6.6869, 4.5802) -> (6.63, 4.6493)
  line L1517 (6.63, 4.6493) -> (6.5674, 4.7321)
  line L1518 (6.5674, 4.7321) -> (6.501, 4.828)
  line L1519 (6.501, 4.828) -> (6.4313, 4.9383)
  line L1520 (6.4313, 4.9383) -> (6.3589, 5.064)
  line L1521 (6.3589, 5.064) -> (6.3226, 5.1319)
  line L1522 (6.3226, 5.1319) -> (6.2584, 5.2612)
  arc A39 (6.4888, 5.5542) -> (6.2584, 5.2612) centre (13.25, 0) ccw
  line L1523 (6.4888, 5.5542) -> (6.6295, 5.5222)
  line L1524 (6.6295, 5.5222) -> (6.7041, 5.5029)
  line L1525 (6.7041, 5.5029) -> (6.8433, 5.4623)
  line L1526 (6.8433, 5.4623) -> (6.967, 5.4205)
  line L1527 (6.967, 5.4205) -> (7.0758, 5.3786)
  line L1528 (7.0758, 5.3786) -> (7.171, 5.3373)
  line L1529 (7.171, 5.3373) -> (7.2516, 5.2982)
  line L1530 (7.2516, 5.2982) -> (7.3208, 5.261)
  line L1531 (7.3208, 5.261) -> (7.3727, 5.2303)
  line L1532 (7.3727, 5.2303) -> (7.446, 5.1839)
  line L1533 (7.446, 5.1839) -> (7.4733, 5.1696)
  line L1534 (7.4733, 5.1696) -> (7.4985, 5.1587)
  line L1535 (7.4985, 5.1587) -> (7.5216, 5.1511)
  line L1536 (7.5216, 5.1511) -> (7.5424, 5.1466)
  line L1537 (7.5424, 5.1466) -> (7.5609, 5.1453)
  line L1538 (7.5609, 5.1453) -> (7.5769, 5.1469)
  line L1539 (7.5769, 5.1469) -> (7.5902, 5.1514)
  line L1540 (7.5902, 5.1514) -> (7.6008, 5.1586)
  line L1541 (7.6008, 5.1586) -> (7.6172, 5.1763)
  line L1542 (7.6172, 5.1763) -> (7.7134, 5.2791)
  line L1543 (7.7134, 5.2791) -> (7.8115, 5.3801)
  line L1544 (7.8115, 5.3801) -> (7.8284, 5.3973)
  line L1545 (7.8284, 5.3973) -> (7.8352, 5.4082)
  line L1546 (7.8352, 5.4082) -> (7.839, 5.4218)
  line L1547 (7.839, 5.4218) -> (7.8399, 5.4378)
  line L1548 (7.8399, 5.4378) -> (7.8376, 5.4562)
  line L1549 (7.8376, 5.4562) -> (7.8322, 5.4768)
  line L1550 (7.8322, 5.4768) -> (7.8235, 5.4995)
  line L1551 (7.8235, 5.4995) -> (7.8114, 5.5242)
  line L1552 (7.8114, 5.5242) -> (7.7958, 5.5508)
  line L1553 (7.7958, 5.5508) -> (7.746, 5.6218)
  line L1554 (7.746, 5.6218) -> (7.7128, 5.6722)
  line L1555 (7.7128, 5.6722) -> (7.6724, 5.7395)
  line L1556 (7.6724, 5.7395) -> (7.6295, 5.8181)
  line L1557 (7.6295, 5.8181) -> (7.5837, 5.9113)
  line L1558 (7.5837, 5.9113) -> (7.5367, 6.018)
  line L1559 (7.5367, 6.018) -> (7.4891, 6.1395)
  line L1560 (7.4891, 6.1395) -> (7.4418, 6.2767)
  line L1561 (7.4418, 6.2767) -> (7.4191, 6.3502)
  line L1562 (7.4191, 6.3502) -> (7.3804, 6.4893)
  arc A40 (7.6621, 6.7334) -> (7.3804, 6.4893) centre (13.25, 0) ccw
  line L1563 (7.6621, 6.7334) -> (7.7943, 6.6753)
  line L1564 (7.7943, 6.6753) -> (7.8638, 6.6423)
  line L1565 (7.8638, 6.6423) -> (7.9928, 6.576)
  line L1566 (7.9928, 6.576) -> (8.1063, 6.5116)
  line L1567 (8.1063, 6.5116) -> (8.2052, 6.4499)
  line L1568 (8.2052, 6.4499) -> (8.291, 6.3913)
  line L1569 (8.291, 6.3913) -> (8.3627, 6.3377)
  line L1570 (8.3627, 6.3377) -> (8.4236, 6.2881)
  line L1571 (8.4236, 6.2881) -> (8.4687, 6.248)
  line L1572 (8.4687, 6.248) -> (8.532, 6.1886)
  line L1573 (8.532, 6.1886) -> (8.556, 6.1694)
  line L1574 (8.556, 6.1694) -> (8.5787, 6.154)
  line L1575 (8.5787, 6.154) -> (8.6, 6.1421)
  line L1576 (8.6, 6.1421) -> (8.6196, 6.1338)
  line L1577 (8.6196, 6.1338) -> (8.6375, 6.129)
  line L1578 (8.6375, 6.129) -> (8.6535, 6.1275)
  line L1579 (8.6535, 6.1275) -> (8.6674, 6.1294)
  line L1580 (8.6674, 6.1294) -> (8.6792, 6.1345)
  line L1581 (8.6792, 6.1345) -> (8.6986, 6.1488)
  line L1582 (8.6986, 6.1488) -> (8.8126, 6.2315)
  line L1583 (8.8126, 6.2315) -> (8.928, 6.3121)
  line L1584 (8.928, 6.3121) -> (8.9478, 6.3258)
  line L1585 (8.9478, 6.3258) -> (8.9565, 6.3353)
  line L1586 (8.9565, 6.3353) -> (8.9629, 6.3479)
  line L1587 (8.9629, 6.3479) -> (8.9667, 6.3634)
  line L1588 (8.9667, 6.3634) -> (8.968, 6.3819)
  line L1589 (8.968, 6.3819) -> (8.9666, 6.4032)
  line L1590 (8.9666, 6.4032) -> (8.9623, 6.4271)
  line L1591 (8.9623, 6.4271) -> (8.9551, 6.4536)
  line L1592 (8.9551, 6.4536) -> (8.9449, 6.4827)
  line L1593 (8.9449, 6.4827) -> (8.9094, 6.5619)
  line L1594 (8.9094, 6.5619) -> (8.8863, 6.6176)
  line L1595 (8.8863, 6.6176) -> (8.8594, 6.6914)
  line L1596 (8.8594, 6.6914) -> (8.8322, 6.7767)
  line L1597 (8.8322, 6.7767) -> (8.8048, 6.8769)
  line L1598 (8.8048, 6.8769) -> (8.7788, 6.9905)
  line L1599 (8.7788, 6.9905) -> (8.7551, 7.1188)
  line L1600 (8.7551, 7.1188) -> (8.7347, 7.2624)
  line L1601 (8.7347, 7.2624) -> (8.7262, 7.339)
  line L1602 (8.7262, 7.339) -> (8.7146, 7.4828)
  arc A41 (9.0374, 7.6692) -> (8.7146, 7.4828) centre (13.25, 0) ccw
  line L1603 (9.0374, 7.6692) -> (9.1562, 7.5872)
  line L1604 (9.1562, 7.5872) -> (9.2182, 7.5416)
  line L1605 (9.2182, 7.5416) -> (9.3324, 7.4521)
  line L1606 (9.3324, 7.4521) -> (9.4316, 7.3674)
  line L1607 (9.4316, 7.3674) -> (9.5171, 7.2881)
  line L1608 (9.5171, 7.2881) -> (9.5901, 7.2143)
  line L1609 (9.5901, 7.2143) -> (9.6504, 7.1481)
  line L1610 (9.6504, 7.1481) -> (9.7008, 7.0878)
  line L1611 (9.7008, 7.0878) -> (9.7376, 7.04)
  line L1612 (9.7376, 7.04) -> (9.7884, 6.9697)
  line L1613 (9.7884, 6.9697) -> (9.8084, 6.9463)
  line L1614 (9.8084, 6.9463) -> (9.8278, 6.9268)
  line L1615 (9.8278, 6.9268) -> (9.8464, 6.9111)
  line L1616 (9.8464, 6.9111) -> (9.8641, 6.8993)
  line L1617 (9.8641, 6.8993) -> (9.8807, 6.8911)
  line L1618 (9.8807, 6.8911) -> (9.8962, 6.8867)
  line L1619 (9.8962, 6.8867) -> (9.9102, 6.8859)
  line L1620 (9.9102, 6.8859) -> (9.9228, 6.8887)
  line L1621 (9.9228, 6.8887) -> (9.9445, 6.899)
  line L1622 (9.9445, 6.899) -> (10.0721, 6.9587)
  line L1623 (10.0721, 6.9587) -> (10.2007, 7.016)
  line L1624 (10.2007, 7.016) -> (10.2227, 7.0257)
  line L1625 (10.2227, 7.0257) -> (10.2331, 7.0333)
  line L1626 (10.2331, 7.0333) -> (10.2417, 7.0445)
  line L1627 (10.2417, 7.0445) -> (10.2484, 7.059)
  line L1628 (10.2484, 7.059) -> (10.2532, 7.0769)
  line L1629 (10.2532, 7.0769) -> (10.2558, 7.0981)
  line L1630 (10.2558, 7.0981) -> (10.2561, 7.1224)
  line L1631 (10.2561, 7.1224) -> (10.2541, 7.1498)
  line L1632 (10.2541, 7.1498) -> (10.2495, 7.1803)
  line L1633 (10.2495, 7.1803) -> (10.2297, 7.2647)
  line L1634 (10.2297, 7.2647) -> (10.2176, 7.3238)
  line L1635 (10.2176, 7.3238) -> (10.2051, 7.4014)
  line L1636 (10.2051, 7.4014) -> (10.1945, 7.4903)
  line L1637 (10.1945, 7.4903) -> (10.1866, 7.5938)
  line L1638 (10.1866, 7.5938) -> (10.1826, 7.7103)
  line L1639 (10.1826, 7.7103) -> (10.1836, 7.8409)
  line L1640 (10.1836, 7.8409) -> (10.1907, 7.9857)
  line L1641 (10.1907, 7.9857) -> (10.1969, 8.0625)
  line L1642 (10.1969, 8.0625) -> (10.2127, 8.2059)
  arc A42 (10.5649, 8.3278) -> (10.2127, 8.2059) centre (13.25, 0) ccw
  line L1643 (10.5649, 8.3278) -> (10.666, 8.2249)
  line L1644 (10.666, 8.2249) -> (10.7183, 8.1683)
  line L1645 (10.7183, 8.1683) -> (10.8135, 8.0589)
  line L1646 (10.8135, 8.0589) -> (10.8949, 7.9569)
  line L1647 (10.8949, 7.9569) -> (10.9638, 7.8628)
  line L1648 (10.9638, 7.8628) -> (11.0216, 7.7765)
  line L1649 (11.0216, 7.7765) -> (11.0683, 7.7001)
  line L1650 (11.0683, 7.7001) -> (11.1063, 7.6314)
  line L1651 (11.1063, 7.6314) -> (11.1334, 7.5775)
  line L1652 (11.1334, 7.5775) -> (11.17, 7.4988)
  line L1653 (11.17, 7.4988) -> (11.1852, 7.4721)
  line L1654 (11.1852, 7.4721) -> (11.2005, 7.4493)
  line L1655 (11.2005, 7.4493) -> (11.2159, 7.4304)
  line L1656 (11.2159, 7.4304) -> (11.231, 7.4154)
  line L1657 (11.231, 7.4154) -> (11.2458, 7.4042)
  line L1658 (11.2458, 7.4042) -> (11.2601, 7.397)
  line L1659 (11.2601, 7.397) -> (11.2737, 7.3935)
  line L1660 (11.2737, 7.3935) -> (11.2866, 7.3939)
  line L1661 (11.2866, 7.3939) -> (11.3099, 7.3999)
  line L1662 (11.3099, 7.3999) -> (11.4464, 7.4344)
  line L1663 (11.4464, 7.4344) -> (11.5836, 7.4663)
  line L1664 (11.5836, 7.4663) -> (11.6071, 7.4716)
  line L1665 (11.6071, 7.4716) -> (11.6187, 7.4772)
  line L1666 (11.6187, 7.4772) -> (11.6292, 7.4865)
  line L1667 (11.6292, 7.4865) -> (11.6386, 7.4995)
  line L1668 (11.6386, 7.4995) -> (11.6467, 7.5162)
  line L1669 (11.6467, 7.5162) -> (11.6532, 7.5365)
  line L1670 (11.6532, 7.5365) -> (11.6582, 7.5603)
  line L1671 (11.6582, 7.5603) -> (11.6614, 7.5876)
  line L1672 (11.6614, 7.5876) -> (11.6626, 7.6183)
  line L1673 (11.6626, 7.6183) -> (11.6591, 7.7051)
  line L1674 (11.6591, 7.7051) -> (11.6584, 7.7654)
  line L1675 (11.6584, 7.7654) -> (11.6608, 7.8439)
  line L1676 (11.6608, 7.8439) -> (11.6673, 7.9332)
  line L1677 (11.6673, 7.9332) -> (11.6791, 8.0364)
  line L1678 (11.6791, 8.0364) -> (11.6972, 8.1515)
  line L1679 (11.6972, 8.1515) -> (11.7229, 8.2795)
  line L1680 (11.7229, 8.2795) -> (11.7573, 8.4204)
  line L1681 (11.7573, 8.4204) -> (11.7779, 8.4946)
  line L1682 (11.7779, 8.4946) -> (11.8205, 8.6324)
  arc A43 (12.1895, 8.6855) -> (11.8205, 8.6324) centre (13.25, 0) ccw
  line L1683 (12.1895, 8.6855) -> (12.2693, 8.5652)
  line L1684 (12.2693, 8.5652) -> (12.3099, 8.4999)
  line L1685 (12.3099, 8.4999) -> (12.3827, 8.3744)
  line L1686 (12.3827, 8.3744) -> (12.4433, 8.2588)
  line L1687 (12.4433, 8.2588) -> (12.4931, 8.1534)
  line L1688 (12.4931, 8.1534) -> (12.5336, 8.0577)
  line L1689 (12.5336, 8.0577) -> (12.5649, 7.9739)
  line L1690 (12.5649, 7.9739) -> (12.5893, 7.8992)
  line L1691 (12.5893, 7.8992) -> (12.6057, 7.8412)
  line L1692 (12.6057, 7.8412) -> (12.6267, 7.757)
  line L1693 (12.6267, 7.757) -> (12.6366, 7.7278)
  line L1694 (12.6366, 7.7278) -> (12.6474, 7.7025)
  line L1695 (12.6474, 7.7025) -> (12.6588, 7.6811)
  line L1696 (12.6588, 7.6811) -> (12.6708, 7.6635)
  line L1697 (12.6708, 7.6635) -> (12.6833, 7.6497)
  line L1698 (12.6833, 7.6497) -> (12.6959, 7.6399)
  line L1699 (12.6959, 7.6399) -> (12.7087, 7.6339)
  line L1700 (12.7087, 7.6339) -> (12.7214, 7.6318)
  line L1701 (12.7214, 7.6318) -> (12.7454, 7.6334)
  line L1702 (12.7454, 7.6334) -> (12.886, 7.6413)
  line L1703 (12.886, 7.6413) -> (13.0267, 7.6468)
  line L1704 (13.0267, 7.6468) -> (13.0508, 7.6475)
  line L1705 (13.0508, 7.6475) -> (13.0632, 7.6508)
  line L1706 (13.0632, 7.6508) -> (13.0753, 7.658)
  line L1707 (13.0753, 7.658) -> (13.087, 7.669)
  line L1708 (13.087, 7.669) -> (13.0981, 7.6838)
  line L1709 (13.0981, 7.6838) -> (13.1084, 7.7025)
  line L1710 (13.1084, 7.7025) -> (13.1177, 7.7249)
  line L1711 (13.1177, 7.7249) -> (13.126, 7.7511)
  line L1712 (13.126, 7.7511) -> (13.1331, 7.7811)
  line L1713 (13.1331, 7.7811) -> (13.1461, 7.8669)
  line L1714 (13.1461, 7.8669) -> (13.1568, 7.9262)
  line L1715 (13.1568, 7.9262) -> (13.174, 8.0029)
  line L1716 (13.174, 8.0029) -> (13.1973, 8.0893)
  line L1717 (13.1973, 8.0893) -> (13.2284, 8.1884)
  line L1718 (13.2284, 8.1884) -> (13.268, 8.2981)
  line L1719 (13.268, 8.2981) -> (13.3174, 8.4189)
  line L1720 (13.3174, 8.4189) -> (13.3778, 8.5507)
  line L1721 (13.3778, 8.5507) -> (13.4121, 8.6197)
  line L1722 (13.4121, 8.6197) -> (13.4801, 8.747)
  arc A44 (13.8524, 8.7292) -> (13.4801, 8.747) centre (13.25, 0) ccw
  line L1723 (13.8524, 8.7292) -> (13.908, 8.5961)
  line L1724 (13.908, 8.5961) -> (13.9355, 8.5242)
  line L1725 (13.9355, 8.5242) -> (13.9832, 8.3872)
  line L1726 (13.9832, 8.3872) -> (14.0209, 8.2622)
  line L1727 (14.0209, 8.2622) -> (14.0499, 8.1493)
  line L1728 (14.0499, 8.1493) -> (14.0714, 8.0477)
  line L1729 (14.0714, 8.0477) -> (14.0864, 7.9594)
  line L1730 (14.0864, 7.9594) -> (14.0962, 7.8815)
  line L1731 (14.0962, 7.8815) -> (14.1013, 7.8214)
  line L1732 (14.1013, 7.8214) -> (14.106, 7.7347)
  line L1733 (14.106, 7.7347) -> (14.1102, 7.7043)
  line L1734 (14.1102, 7.7043) -> (14.116, 7.6774)
  line L1735 (14.116, 7.6774) -> (14.1232, 7.6541)
  line L1736 (14.1232, 7.6541) -> (14.1316, 7.6346)
  line L1737 (14.1316, 7.6346) -> (14.1412, 7.6187)
  line L1738 (14.1412, 7.6187) -> (14.1518, 7.6067)
  line L1739 (14.1518, 7.6067) -> (14.1632, 7.5984)
  line L1740 (14.1632, 7.5984) -> (14.1753, 7.594)
  line L1741 (14.1753, 7.594) -> (14.1992, 7.5909)
  line L1742 (14.1992, 7.5909) -> (14.3387, 7.5721)
  line L1743 (14.3387, 7.5721) -> (14.4779, 7.5508)
  line L1744 (14.4779, 7.5508) -> (14.5017, 7.547)
  line L1745 (14.5017, 7.547) -> (14.5145, 7.5479)
  line L1746 (14.5145, 7.5479) -> (14.5278, 7.5526)
  line L1747 (14.5278, 7.5526) -> (14.5413, 7.5612)
  line L1748 (14.5413, 7.5612) -> (14.555, 7.5737)
  line L1749 (14.555, 7.5737) -> (14.5686, 7.5901)
  line L1750 (14.5686, 7.5901) -> (14.5821, 7.6104)
  line L1751 (14.5821, 7.6104) -> (14.5952, 7.6345)
  line L1752 (14.5952, 7.6345) -> (14.6078, 7.6626)
  line L1753 (14.6078, 7.6626) -> (14.6368, 7.7444)
  line L1754 (14.6368, 7.7444) -> (14.6585, 7.8006)
  line L1755 (14.6585, 7.8006) -> (14.6899, 7.8727)
  line L1756 (14.6899, 7.8727) -> (14.7291, 7.9531)
  line L1757 (14.7291, 7.9531) -> (14.7785, 8.0445)
  line L1758 (14.7785, 8.0445) -> (14.8381, 8.1447)
  line L1759 (14.8381, 8.1447) -> (14.9094, 8.254)
  line L1760 (14.9094, 8.254) -> (14.9938, 8.372)
  line L1761 (14.9938, 8.372) -> (15.0404, 8.4332)
  line L1762 (15.0404, 8.4332) -> (15.1313, 8.5454)
  arc A45 (15.4935, 8.4575) -> (15.1313, 8.5454) centre (13.25, 0) ccw
  line L1763 (15.4935, 8.4575) -> (15.5229, 8.3162)
  line L1764 (15.5229, 8.3162) -> (15.5364, 8.2404)
  line L1765 (15.5364, 8.2404) -> (15.5572, 8.0968)
  line L1766 (15.5572, 8.0968) -> (15.5706, 7.967)
  line L1767 (15.5706, 7.967) -> (15.5777, 7.8506)
  line L1768 (15.5777, 7.8506) -> (15.5796, 7.7468)
  line L1769 (15.5796, 7.7468) -> (15.5776, 7.6573)
  line L1770 (15.5776, 7.6573) -> (15.5725, 7.5789)
  line L1771 (15.5725, 7.5789) -> (15.5661, 7.519)
  line L1772 (15.5661, 7.519) -> (15.5544, 7.433)
  line L1773 (15.5544, 7.433) -> (15.5527, 7.4022)
  line L1774 (15.5527, 7.4022) -> (15.5533, 7.3747)
  line L1775 (15.5533, 7.3747) -> (15.5559, 7.3506)
  line L1776 (15.5559, 7.3506) -> (15.5605, 7.3298)
  line L1777 (15.5605, 7.3298) -> (15.567, 7.3124)
  line L1778 (15.567, 7.3124) -> (15.5751, 7.2986)
  line L1779 (15.5751, 7.2986) -> (15.5847, 7.2883)
  line L1780 (15.5847, 7.2883) -> (15.5957, 7.2816)
  line L1781 (15.5957, 7.2816) -> (15.6186, 7.2741)
  line L1782 (15.6186, 7.2741) -> (15.7521, 7.2293)
  line L1783 (15.7521, 7.2293) -> (15.8847, 7.182)
  line L1784 (15.8847, 7.182) -> (15.9073, 7.1738)
  line L1785 (15.9073, 7.1738) -> (15.9201, 7.1722)
  line L1786 (15.9201, 7.1722) -> (15.934, 7.1743)
  line L1787 (15.934, 7.1743) -> (15.949, 7.1802)
  line L1788 (15.949, 7.1802) -> (15.9647, 7.1899)
  line L1789 (15.9647, 7.1899) -> (15.9812, 7.2034)
  line L1790 (15.9812, 7.2034) -> (15.9983, 7.2207)
  line L1791 (15.9983, 7.2207) -> (16.0157, 7.242)
  line L1792 (16.0157, 7.242) -> (16.0334, 7.2672)
  line L1793 (16.0334, 7.2672) -> (16.0773, 7.342)
  line L1794 (16.0773, 7.342) -> (16.1094, 7.3931)
  line L1795 (16.1094, 7.3931) -> (16.1538, 7.4579)
  line L1796 (16.1538, 7.4579) -> (16.2075, 7.5295)
  line L1797 (16.2075, 7.5295) -> (16.2733, 7.6099)
  line L1798 (16.2733, 7.6099) -> (16.3508, 7.697)
  line L1799 (16.3508, 7.697) -> (16.4415, 7.7908)
  line L1800 (16.4415, 7.7908) -> (16.5467, 7.8907)
  line L1801 (16.5467, 7.8907) -> (16.6041, 7.942)
  line L1802 (16.6041, 7.942) -> (16.7145, 8.0349)
  arc A46 (17.0536, 7.88) -> (16.7145, 8.0349) centre (13.25, 0) ccw
  line L1803 (17.0536, 7.88) -> (17.0557, 7.7357)
  line L1804 (17.0557, 7.7357) -> (17.0545, 7.6588)
  line L1805 (17.0545, 7.6588) -> (17.0479, 7.5139)
  line L1806 (17.0479, 7.5139) -> (17.0364, 7.3838)
  line L1807 (17.0364, 7.3838) -> (17.0214, 7.2683)
  line L1808 (17.0214, 7.2683) -> (17.0036, 7.1659)
  line L1809 (17.0036, 7.1659) -> (16.9847, 7.0784)
  line L1810 (16.9847, 7.0784) -> (16.9649, 7.0024)
  line L1811 (16.9649, 7.0024) -> (16.9472, 6.9448)
  line L1812 (16.9472, 6.9448) -> (16.9194, 6.8625)
  line L1813 (16.9194, 6.8625) -> (16.912, 6.8327)
  line L1814 (16.912, 6.8327) -> (16.9073, 6.8056)
  line L1815 (16.9073, 6.8056) -> (16.9054, 6.7813)
  line L1816 (16.9054, 6.7813) -> (16.906, 6.76)
  line L1817 (16.906, 6.76) -> (16.909, 6.7418)
  line L1818 (16.909, 6.7418) -> (16.9143, 6.7266)
  line L1819 (16.9143, 6.7266) -> (16.9218, 6.7147)
  line L1820 (16.9218, 6.7147) -> (16.9314, 6.7061)
  line L1821 (16.9314, 6.7061) -> (16.9524, 6.6944)
  line L1822 (16.9524, 6.6944) -> (17.075, 6.6251)
  line L1823 (17.075, 6.6251) -> (17.1963, 6.5536)
  line L1824 (17.1963, 6.5536) -> (17.217, 6.5412)
  line L1825 (17.217, 6.5412) -> (17.2292, 6.5373)
  line L1826 (17.2292, 6.5373) -> (17.2433, 6.5367)
  line L1827 (17.2433, 6.5367) -> (17.259, 6.5397)
  line L1828 (17.259, 6.5397) -> (17.2764, 6.5462)
  line L1829 (17.2764, 6.5462) -> (17.2951, 6.5563)
  line L1830 (17.2951, 6.5563) -> (17.3151, 6.5701)
  line L1831 (17.3151, 6.5701) -> (17.3363, 6.5877)
  line L1832 (17.3363, 6.5877) -> (17.3584, 6.6091)
  line L1833 (17.3584, 6.6091) -> (17.4157, 6.6742)
  line L1834 (17.4157, 6.6742) -> (17.4568, 6.7184)
  line L1835 (17.4568, 6.7184) -> (17.5128, 6.7736)
  line L1836 (17.5128, 6.7736) -> (17.5791, 6.8337)
  line L1837 (17.5791, 6.8337) -> (17.6588, 6.9002)
  line L1838 (17.6588, 6.9002) -> (17.7514, 6.9711)
  line L1839 (17.7514, 6.9711) -> (17.8583, 7.046)
  line L1840 (17.8583, 7.046) -> (17.9804, 7.1242)
  line L1841 (17.9804, 7.1242) -> (18.0465, 7.1637)
  line L1842 (18.0465, 7.1637) -> (18.1725, 7.234)
  arc A47 (18.4762, 7.0178) -> (18.1725, 7.234) centre (13.25, 0) ccw
  line L1843 (18.4762, 7.0178) -> (18.4509, 6.8757)
  line L1844 (18.4509, 6.8757) -> (18.4352, 6.8003)
  line L1845 (18.4352, 6.8003) -> (18.4013, 6.6593)
  line L1846 (18.4013, 6.6593) -> (18.3654, 6.5338)
  line L1847 (18.3654, 6.5338) -> (18.3287, 6.4232)
  line L1848 (18.3287, 6.4232) -> (18.292, 6.326)
  line L1849 (18.292, 6.326) -> (18.2568, 6.2437)
  line L1850 (18.2568, 6.2437) -> (18.2229, 6.1728)
  line L1851 (18.2229, 6.1728) -> (18.1947, 6.1196)
  line L1852 (18.1947, 6.1196) -> (18.1518, 6.0441)
  line L1853 (18.1518, 6.0441) -> (18.1389, 6.0162)
  line L1854 (18.1389, 6.0162) -> (18.1292, 5.9904)
  line L1855 (18.1292, 5.9904) -> (18.1227, 5.967)
  line L1856 (18.1227, 5.967) -> (18.1192, 5.946)
  line L1857 (18.1192, 5.946) -> (18.1188, 5.9275)
  line L1858 (18.1188, 5.9275) -> (18.1211, 5.9116)
  line L1859 (18.1211, 5.9116) -> (18.1262, 5.8985)
  line L1860 (18.1262, 5.8985) -> (18.134, 5.8882)
  line L1861 (18.134, 5.8882) -> (18.1524, 5.8727)
  line L1862 (18.1524, 5.8727) -> (18.2597, 5.7815)
  line L1863 (18.2597, 5.7815) -> (18.3653, 5.6883)
  line L1864 (18.3653, 5.6883) -> (18.3832, 5.6723)
  line L1865 (18.3832, 5.6723) -> (18.3945, 5.6661)
  line L1866 (18.3945, 5.6661) -> (18.4082, 5.6629)
  line L1867 (18.4082, 5.6629) -> (18.4242, 5.6628)
  line L1868 (18.4242, 5.6628) -> (18.4425, 5.6659)
  line L1869 (18.4425, 5.6659) -> (18.4628, 5.6723)
  line L1870 (18.4628, 5.6723) -> (18.4851, 5.6821)
  line L1871 (18.4851, 5.6821) -> (18.5092, 5.6953)
  line L1872 (18.5092, 5.6953) -> (18.5349, 5.7121)
  line L1873 (18.5349, 5.7121) -> (18.6036, 5.7653)
  line L1874 (18.6036, 5.7653) -> (18.6523, 5.8008)
  line L1875 (18.6523, 5.8008) -> (18.7176, 5.8444)
  line L1876 (18.7176, 5.8444) -> (18.7941, 5.8909)
  line L1877 (18.7941, 5.8909) -> (18.885, 5.9411)
  line L1878 (18.885, 5.9411) -> (18.9893, 5.9932)
  line L1879 (18.9893, 5.9932) -> (19.1084, 6.0465)
  line L1880 (19.1084, 6.0465) -> (19.2432, 6.1002)
  line L1881 (19.2432, 6.1002) -> (19.3156, 6.1265)
  line L1882 (19.3156, 6.1265) -> (19.4526, 6.1717)